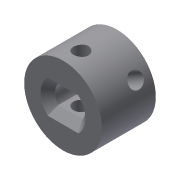
# Autodesk Inventor part: 30_Coupling_Screw_28BYJ_M3
Saved by Autodesk Inventor 2019.4 (Build 234330000, 330)
## iProperties
Created: 2019-05-13
Part Number: 30_Coupling_Screw_28BYJ_M3
Material: Generic
Document SubType Name: Modeling
Designer: diederichbenedict
Density: 1 g/cm^3
Appearance: Default
Author: diederichbenedict
Autodesk Inventor part; units mm, degrees
ref_plane "YZ Plane" through (0, 0, 0) normal (1, 0, 0) x (0, 1, 0)
ref_plane "XZ Plane" through (0, 0, 0) normal (0, 1, 0) x (-1, 0, 0)
sketch "Sketch1" plane through (0, 0, 0) normal (0, 0, 1) x (1, 0, 0)
  line L0 (0.8467, -0.7217) -> (0.8467, 0.7217) construction
  line L1 (0.8467, 0.7217) -> (2.0967, 1.4434) construction
  line L2 (2.0967, 1.4434) -> (3.3467, 0.7217) construction
  line L3 (3.3467, 0.7217) -> (3.3467, -0.7217) construction
  line L4 (3.3467, -0.7217) -> (2.0967, -1.4434) construction
  line L5 (2.0967, -1.4434) -> (0.8467, -0.7217) construction
  circle A0 centre (2.0967, 0) radius 2.45 construction
  line L6 (4.8467, -1.5877) -> (3.4717, -2.3816) construction
  line L7 (15.0967, 3) -> (15.0967, -3) construction
  line L8 (-10.9033, 3) -> (-10.9033, -3) construction
  line L9 (-0.6533, 0) -> (-0.6533, 1.5877) construction
  circle A1 centre (2.0967, 0) radius 5
  circle A2 centre (2.0967, 0) radius 1.7 projected
  line L10 (-10.9033, -3) -> (15.0967, -3) projected
  line L11 (-10.9033, 3) -> (15.0967, 3) projected
  circle A3 centre (2.0967, 0) radius 2.7
  circle A4 centre (2.0967, 0) radius 6.5
  circle A5 centre (2.0967, 0) radius 2.75
  point P0 (0.4719, -0.5)
  point P1 (3.7215, -0.5)
  dimension "d10" = 5.4
  dimension "d13" = 13
  constraints: 4 centre point, 2 coincident, 2 other
  measures "d10" diameter of A3
  measures "d13" diameter of A4
ref_plane "Work Plane1" through (-20.8033, -6.3, -5.9) normal (0, 0, 1) x (1, 0, 0)
extrude "Extrusion1" add sketch "Sketch1" against normal blind 4 contours A1 L10 L11 | A1 L11 A4 L10 | L11 A1 | A1 L11 A4 | L10 A4 A1 | A1 L10 | A1 L10 A4 L11 | A5
sketch "Sketch2" plane through (2.0967, 0, 0) normal (0, 0, 1) x (1, 0, 0)
  line L0 (-2, 1.5) -> (2, 1.5) construction
  arc A0 (2.5, 0) -> (2, 1.5) centre (0, 0) ccw construction
  arc A1 (-2, 1.5) -> (-2.5, 0) centre (0, 0) ccw construction
  line L1 (2, -1.5) -> (-2, -1.5) construction
  arc A2 (-2.5, 0) -> (2.5, 0) centre (0, 0) ccw construction
  line L2 (2.0248, 1.55) -> (-2.0248, 1.55) construction
  arc A3 (-2.0248, 1.55) -> (-2.55, 0) centre (0, 0) ccw construction
  arc A4 (-2.55, 0) -> (2.55, 0) centre (0, 0) ccw construction
  arc A5 (2.55, 0) -> (2.0248, 1.55) centre (0, 0) ccw construction
  line L3 (-2.0248, 1.55) -> (2.0248, 1.55) construction
  line L4 (-2.0248, 1.55) -> (2.0248, 1.55)
  line L5 (-2.0248, -1.55) -> (2.0248, -1.55)
  arc A6 (-2.0248, 1.55) -> (-2.0248, -1.55) centre (0, 0) ccw
  arc A7 (2.0248, -1.55) -> (2.0248, 1.55) centre (0, 0) ccw
  circle A8 centre (0, 0) radius 6.5 projected
  point P0 (-2.0967, 0)
  dimension "d11" = 3.1
  dimension "d12" = 2.55
  constraints: 14 point on circle, 8 end point, 5 centre point, 2 equal length, 1 horizontal, 3 other
  measures "d11" distance between parallel lines of L2 L5
  measures "d12" radius of A6
extrude "Extrusion2" add sketch "Sketch2" along normal blind 5
chamfer "Chamfer1" distance 1.2 angle 45 4 edges at (2.0967, 1.55, 5) (-0.4533, 0, 5) (2.0967, -1.55, 5) (4.6467, 0, 5)
sketch "Sketch3" plane through (0, 0, 0) normal (0, 1, 0) x (-1, 0, 0)
  line L0 (-4.6467, 0) -> (-4.6467, 3.8) projected
  line L1 (0.4533, 0) -> (0.4533, 3.8) projected
  line L2 (-8.5967, -4) -> (4.4033, -4) projected
  circle A0 centre (-2.0967, -1.5) radius 1.25
  line L3 (-8.5967, -4) -> (4.4033, -4) projected
  point P0 (0, 0)
  point P1 (-8.5967, 0)
  point P2 (4.4033, 0)
  dimension "d14" = 2.5
  dimension "d15" = 2.5
  constraints: 1 centre point
  measures "d14" diameter of A0
  measures "d15" distance from line of A0.centre L3
extrude "Extrusion3" cut sketch "Sketch3" against normal blind 10
pattern_circular "Circular Pattern1" count 3 over 360 about axis through (2.0967, 0, 0) along (0, 0, -1) of "Extrusion3"
sketch "Sketch4" plane through (0.0718, -1.55, 0) normal (0, 1, 0) x (1, 0, 0)
  line L0 (0, -3.8) -> (4.0497, -3.8) projected
  line L1 (-4.4752, -5) -> (8.5248, -5) projected
  line L2 (8.5248, 4) -> (-4.4752, 4) projected
  line L3 (4.0497, -3.8) -> (0, -3.8) projected
  line L4 (4.0497, 0) -> (4.0497, -3.8) projected
  line L5 (0, 0) -> (4.0497, 0) projected
  line L6 (0, 0) -> (0, -3.8) projected
  circle A0 centre (2.0248, -2.0248) radius 2.0248
  point P0 (-0.0718, 0)
  point P1 (8.1739, 1.5)
  point P2 (-2.8742, 1.5)
  point P3 (0.7748, 1.5)
  constraints: 3 tangent, 1 centre point, 3 other
hole "Hole1" at (2.0967, -1.55, 2.0248) direction (0, -1, 0) diameter 2.5 end through all both
body "Solid1"
